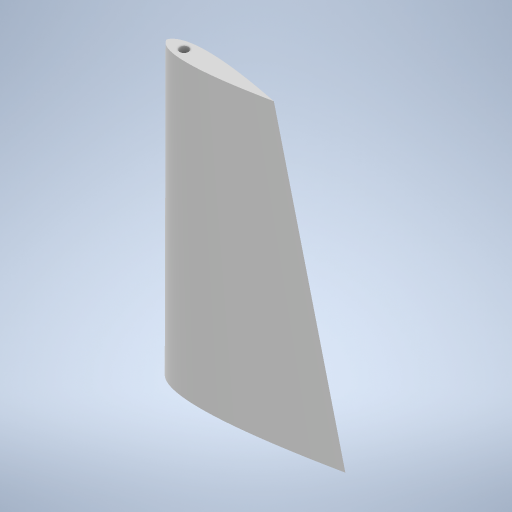
# Autodesk Inventor part: mb_sail
Saved by Autodesk Inventor 2023 (Build 270158000, 158)
## iProperties
Created: 2023-01-28
Part Number: mb_sail
Material: Generisch
Document SubType Name: Modeling
Designer: georg
Density: 1 g/cm^3
Appearance: Vorgabe
Author: georg
Autodesk Inventor part; units mm, degrees
ref_plane "YZ Plane" through (0, 0, 0) normal (1, 0, 0) x (0, 1, 0)
ref_plane "XY Plane" through (0, 0, 0) normal (0, 0, 1) x (1, 0, 0)
sketch "ground" plane through (0, 0, 0) normal (0, 1, 0) x (-1, 0, 0)
  line L0 (483.3377, 0) -> (445.9963, 94.5527) construction
  line L1 (445.9963, 94.5527) -> (-16.6623, 0) construction
  spline S0 degree 2 poles (483.3377, 0) (445.9963, 94.5527) (-16.6623, 0) knots 1 1 1 2 2 2
  line L2 (483.3377, 0) -> (-16.6623, 0)
  point P0 (0, 0)
  dimension "d0" = 500
  dimension "d21" = 100
  dimension "d22" = 68.45
  constraints: 3 end point, 1 horizontal, 3 other
  measures "d0" distance of L0.start L1.end
  measures "d21" angle of L0 L1
  measures "d22" angle of L2 L0
ref_plane "Arbeitsebene1" through (0, 800, 0) normal (0, 1, 0) x (-1, 0, 0)
sketch "Skizze3" plane through (0, 800, 0) normal (0, 1, 0) x (-1, 0, 0)
  line L0 (483.3697, 0) -> (460.9649, 56.7316) construction
  line L1 (460.9649, 56.7316) -> (183.3697, 0) construction
  spline S0 degree 2 poles (483.3697, 0) (460.9649, 56.7316) (183.3697, 0) knots 1 1 1 2 2 2
  line L2 (483.3697, 0) -> (183.3697, 0)
  point P0 (0, 0)
  dimension "d27" = 300
  dimension "d28" = 100
  dimension "d29" = 68.45
  constraints: 3 end point, 1 horizontal, 3 other
  measures "d27" distance of L0.start L1.end
  measures "d28" angle of L0 L1
  measures "d29" angle of L2 L0
sketch "Skizze5" plane through (0, 800, 0) normal (0, 1, 0) x (-1, 0, 0)
  circle A0 centre (434.5806, 0) radius 12.3812
  point P0 (0, 0)
  constraints: 1 centre point
loft "Erhebung2" add profiles "ground", "Skizze3"
mirror "Spiegeln2" about plane through (16.6623, 0, 0) normal (0, 0, -1) of "Erhebung2"
hole "Bohrung1" at (-434.5806, 800, 0) direction (0, -1, 0) diameter 25 end through all
